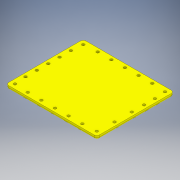
# Autodesk Inventor part: back_lid
Saved by Autodesk Inventor 2018 (Build 220112000, 112)
## iProperties
Created: 2019-07-25
Part Number: back_lid
Material: Generic
Document SubType Name: Modeling
Designer: ZEUSLAP
Density: 1 g/cm^3
Appearance: Default
Author: ZEUSLAP
## iProperties of the stored document back_lid_generic_3DPrint.ipt
Created: 2019-09-09
Part Number: back_lid_generic_3DPrint
Material: Generic
Document SubType Name: Modeling
Designer: ZEUSLAP
Density: 1 g/cm^3
Appearance: Default
Author: ZEUSLAP
Autodesk Inventor part; units mm, degrees
ref_plane "YZ Plane" through (0, 0, 0) normal (1, 0, 0) x (0, 1, 0)
ref_plane "XZ Plane" through (0, 0, 0) normal (0, 1, 0) x (-1, 0, 0)
ref_plane "XY Plane" through (0, 0, 0) normal (0, 0, 1) x (1, 0, 0)
sketch "lid shape" plane through (0, 0, 0) normal (0, 0, 1) x (1, 0, 0)
  line L0 (-50, 42.5) -> (50, 42.5)
  line L1 (50, 42.5) -> (50, -42.5)
  line L2 (50, -42.5) -> (-50, -42.5)
  line L3 (-50, -42.5) -> (-50, 42.5)
  line L4 (40, 32.5) -> (-40, 32.5)
  line L5 (-40, 32.5) -> (-40, -32.5)
  line L6 (-40, -32.5) -> (40, -32.5)
  line L7 (40, -32.5) -> (40, 32.5)
  point P0 (0, 0)
  point P1 (0, -42.5)
  point P2 (50, 0)
  dimension "d0" = 100
  dimension "d1" = 85
  dimension "d2" = 10
  constraints: 16 end point, 4 parallel, 2 midpoint, 2 perpendicular, 1 horizontal, 1 horizontal alignment, 1 vertical alignment, 3 other
  measures "d0" distance of L0.start L0.end
  measures "d1" distance of L0.end L1.end
  measures "d2" distance between parallel lines of L0 L4
extrude "lid bulk" add sketch "lid shape" along normal blind 2 contours L0 L1 L2 L3 | L7 L6 L5 L4
extrude "lip" add sketch "lid shape" against normal blind 2
sketch "m3 nuts" plane through (0, 0, 0) normal (0, 0, 1) x (1, 0, 0)
  line L0 (50, 42.5) -> (-50, 42.5)
  line L1 (-50, 42.5) -> (-50, -42.5)
  line L2 (-50, -42.5) -> (50, -42.5)
  line L3 (50, -42.5) -> (50, 42.5)
  circle A0 centre (-45, 37.5) radius 1.5
  circle A1 centre (45, 37.5) radius 1.5
  circle A2 centre (45, -37.5) radius 1.5
  circle A3 centre (-45, -37.5) radius 1.5
  circle A4 centre (-30, 38.5) radius 1.5
  circle A5 centre (-15, 38.5) radius 1.5
  circle A6 centre (15, 38.5) radius 1.5
  circle A7 centre (30, 38.5) radius 1.5
  circle A8 centre (0, 38.5) radius 1.5
  circle A9 centre (-30, -38.5) radius 1.5
  circle A10 centre (-15, -38.5) radius 1.5
  circle A11 centre (0, -38.5) radius 1.5
  circle A12 centre (15, -38.5) radius 1.5
  circle A13 centre (30, -38.5) radius 1.5
  circle A14 centre (45, 37.5) radius 3.5
  circle A15 centre (30, 38.5) radius 3.5
  circle A16 centre (15, 38.5) radius 3.5
  circle A17 centre (0, 38.5) radius 3.5
  circle A18 centre (-15, 38.5) radius 3.5
  circle A19 centre (-30, 38.5) radius 3.5
  circle A20 centre (-45, 37.5) radius 3.5
  circle A21 centre (-45, -37.5) radius 3.5
  circle A22 centre (-30, -38.5) radius 3.5
  circle A23 centre (-15, -38.5) radius 3.5
  circle A24 centre (0, -38.5) radius 3.5
  circle A25 centre (15, -38.5) radius 3.5
  circle A26 centre (30, -38.5) radius 3.5
  circle A27 centre (45, -37.5) radius 3.5
  line L4 (0, -70.7711) -> (0, 85.4477) construction
  circle A28 centre (46, 0) radius 1.5
  circle A29 centre (46, -19) radius 1.5
  circle A30 centre (-46, -12.5) radius 1.5
  circle A31 centre (46, 25.5) radius 1.5
  circle A32 centre (46, 13.5) radius 1.5
  circle A33 centre (-46, 25) radius 1.5
  circle A34 centre (-46, 12.5) radius 1.5
  circle A35 centre (-46, 0) radius 1.5
  circle A36 centre (-46, -25) radius 1.5
  circle A37 centre (46, 25.5) radius 3.5
  circle A38 centre (46, 13.5) radius 3.5
  circle A39 centre (46, 0) radius 3.5
  circle A40 centre (46, -19) radius 3.5
  circle A41 centre (-46, -25) radius 3.5
  circle A42 centre (-46, -12.5) radius 3.5
  circle A43 centre (-46, 0) radius 3.5
  circle A44 centre (-46, 12.5) radius 3.5
  circle A45 centre (-46, 25) radius 3.5
  line L5 (76.7842, 0) -> (-92.3219, 0) construction
  line L6 (46, 0) -> (46, -19) construction
  point P0 (0, 0)
  point P1 (0, 0)
  point P2 (0, 0)
  point P3 (46, -9.5)
  dimension "d7" = 3
  dimension "d8" = 5
  dimension "d9" = 5
  dimension "d11" = 4
  dimension "d12" = 15
  dimension "d13" = 15
  dimension "d14" = 15
  dimension "d30" = 7
  dimension "d31" = 18.5
  dimension "d32" = 12.5
  dimension "d33" = 12.5
  dimension "d34" = 19
  dimension "d35" = 12.5
  dimension "d36" = 12
  dimension "d37" = 12
  dimension "d38" = 13.5
  dimension "d41" = 52
  dimension "d42" = 100
  dimension "d43" = 85
  constraints: 48 coincident, 46 centre point, 28 equal radius, 14 end point, 3 vertical, 2 horizontal, 2 horizontal alignment, 2 point on line, 1 midpoint, 5 other
  measures "d7" diameter of A0
  measures "d8" distance from line of L0 A0.centre
  measures "d9" distance from line of L1 A0.centre
  measures "d11" distance from line of L0 A4.centre
  measures "d12" horizontal distance of A4.centre A0.centre
  measures "d13" distance of A5.centre A4.centre
  measures "d14" distance of A8.centre A5.centre
  measures "d30" diameter of A14
  measures "d31" vertical distance of A2.centre A29.centre
  measures "d32" vertical distance of A36.centre A3.centre
  measures "d33" distance of point (-46, -12.5) A41.centre
  measures "d34" distance of A29.centre A28.centre
  measures "d35" distance of A35.centre point (-46, -12.5)
  measures "d36" vertical distance of A1.centre point (46, 25.5)
  measures "d37" distance of A32.centre point (46, 25.5)
  measures "d38" distance of A28.centre A32.centre
  measures "d41" distance from line of L0 point (46, -9.5)
  measures "d42" distance of L0.start L0.end
  measures "d43" distance of L2.end L0.start
extrude "m3 bolt holes" cut sketch "m3 nuts" along normal through all both and the other way through all contours A0 | A1 | A2 | A3 | A4 | A5 | A6 | A7 | A8 | A9 | A10 | A11 | A12 | A13 | A28 | A29 | A30 | A31 | A32 | A33 | A34 | A35 | A36
extrude "m3 bolt head recesses" cut sketch "m3 nuts" against normal up to surface (2 mm away) contours A14 | A15 | A16 | A17 | A18 | A19 | A20 | A21 | A22 | A23 | A24 | A25 | A26 | A27 | A37 | A38 | A39 | A40 | A41 | A42 | A43 | A44 | A45
fillet "2mm filet" radius 2 8 edges at (40, 0, -2) (40, 0, 0) (-40, 0, -2) (-40, 0, 0) (50, 0, -2) (0, 42.5, -2) (-50, 0, -2) (0, -42.5, -2)
fillet "4mm filet" radius 3 8 edges at (-49.4142, 41.9142, -1.4142) (-50, 42.5, 1) (49.4142, 41.9142, -1.4142) (50, 42.5, 1) (49.4142, -41.9142, -1.4142) (50, -42.5, 1) (-49.4142, -41.9142, -1.4142) (-50, -42.5, 1)
equation "\"d13\" = d12"
equation "\"d14\" = d12"
equation "\"d33\" = d32"
equation "\"d37\" = d36"
body "Solid1"
